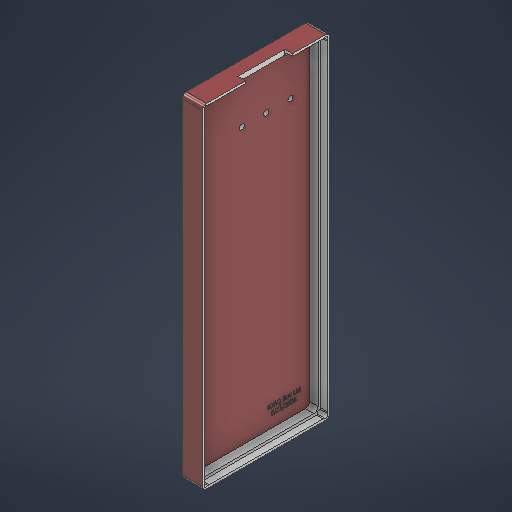
# Autodesk Inventor part: cDAQ_Lid_Box
Saved by Autodesk Inventor 2027 (Build 310192000, 192)
## iProperties
Created: 2026-05-08
Part Number: cDAQ_Lid_Box
Material: Generic
Document SubType Name: Modeling
Designer: giese
Density: 1 g/cm^3
Appearance: Default
Author: giese
Autodesk Inventor part; units mm, degrees
(part 1 of 2)
ref_plane "YZ Plane" through (0, 0, 0) normal (1, 0, 0) x (0, 1, 0)
ref_plane "XZ Plane" through (0, 0, 0) normal (0, 1, 0) x (-1, 0, 0)
ref_plane "XY Plane" through (0, 0, 0) normal (0, 0, 1) x (1, 0, 0)
sketch "Sketch1" plane through (0, 0, 0) normal (1, 0, 0) x (0, 1, 0)
  line L0 (50.7569, 48.4212) -> (-202.6081, 48.4212)
  line L1 (-202.6081, 48.4212) -> (-202.6081, -48.0988)
  line L2 (-202.6081, -48.0988) -> (50.7569, -48.0988)
  line L3 (50.7569, -48.0988) -> (50.7569, 48.4212)
  point P0 (0, 0)
  dimension "d0" = 96.52
  dimension "d1" = 253.365
  constraints: 8 end point, 2 parallel, 1 horizontal, 1 perpendicular
  measures "d0" distance of L2.end L0.start
  measures "d1" distance of L0.start L0.end
extrude "Extrusion1" add sketch "Sketch1" along normal blind 15.24
sketch "Sketch2" plane through (15.24, 0, 0) normal (1, 0, 0) x (0, 0, -1)
  line L0 (-44.6112, 46.9469) -> (44.2888, 46.9469)
  line L1 (44.2888, 46.9469) -> (44.2888, -198.7981)
  line L2 (44.2888, -198.7981) -> (-44.6112, -198.7981)
  line L3 (-44.6112, -198.7981) -> (-44.6112, 46.9469)
  line L4 (-48.4212, 50.7569) -> (-48.4212, -202.6081) projected
  line L5 (-48.4212, -202.6081) -> (48.0988, -202.6081) projected
  point P0 (0, 0)
  dimension "d4" = 88.9
  dimension "d5" = 245.745
  dimension "d6" = 3.81
  dimension "d7" = 3.81
  constraints: 8 end point, 2 parallel, 1 horizontal, 1 perpendicular
  measures "d4" distance of L0.start L0.end
  measures "d5" distance of L0.end L1.end
  measures "d6" distance between parallel lines of L4 L3
  measures "d7" distance between parallel lines of L5 L2
extrude "Extrusion2" cut sketch "Sketch2" against normal blind 11.43
sketch "Sketch3" plane through (0, 0, 0) normal (-1, 0, 0) x (0, 0, 1)
  circle A0 centre (-29.8108, 10.5233) radius 2
  line L0 (-48.0988, -202.6081) -> (-48.0988, 50.7569) projected
  line L1 (-48.0988, 50.7569) -> (48.4212, 50.7569) projected
  circle A1 centre (-11.312, 10.5233) radius 2
  circle A2 centre (7.1869, 10.5233) radius 2
  point P0 (0, 0)
  dimension "d10" = 18.288
  dimension "d11" = 40.2336
  dimension "d12" = 40.2336
  dimension "d13" = 18.4988
  dimension "d14" = 4
  dimension "d15" = 4
  dimension "d16" = 40.2336
  dimension "d17" = 18.4988
  dimension "d18" = 36.9976
  dimension "d21" = 4
  constraints: 3 centre point
  measures "d10" distance from line of L0 A0.centre
  measures "d11" distance from line of L1 A0.centre
  measures "d12" distance from line of L1 A1.centre
  measures "d13" distance of A0.centre A1.centre
  measures "d14" diameter of A1
  measures "d15" diameter of A2
  measures "d16" distance from line of L1 A2.centre
  measures "d17" distance of A1.centre A2.centre
  measures "d18" distance of A0.centre A2.centre
  measures "d21" diameter of A0
extrude "Extrusion3" cut sketch "Sketch3" against normal blind 3.81
sketch "Sketch6" plane through (0, 50.7569, 48.4212) normal (0, 1, 0) x (1, 0, 0)
  line L0 (15.24, 3.81) -> (15.24, 92.71) projected
  line L1 (9.4234, 32.7559) -> (15.24, 32.7559)
  line L2 (15.24, 32.7559) -> (15.24, 68.326)
  line L3 (15.24, 68.326) -> (9.4234, 68.326)
  line L4 (9.4234, 68.326) -> (9.4234, 32.7559)
  line L5 (0, 96.52) -> (15.24, 96.52) projected
  point P0 (0, 48.4212)
  point P1 (12.3317, 68.326)
  point P2 (12.3317, 32.7559)
  dimension "d30" = 5.8166
  dimension "d31" = 35.5701
  dimension "d32" = 28.194
  constraints: 8 end point, 2 midpoint, 2 parallel, 1 horizontal, 1 perpendicular, 1 point on line
  measures "d30" distance between parallel lines of L0 L4
  measures "d31" distance of point (12.332, 68.326) point (12.332, 32.756)
  measures "d32" distance between parallel lines of L5 L3
extrude "Extrusion5" cut sketch "Sketch6" against normal blind 3.81
fillet "Fillet1" radius 3.175 4 edges at (7.62, 50.7569, -48.0988) (7.62, 50.7569, 48.4212) (7.62, -202.6081, 48.4212) (7.62, -202.6081, -48.0988)
sketch "Sketch7" plane through (15.24, 0, 0) normal (1, 0, 0) x (0, 0, -1)
  line L0 (-44.6112, -198.7981) -> (-44.6112, 46.9469) projected
  line L1 (-44.6112, 46.9469) -> (-42.3252, 46.9469)
  line L2 (-42.3252, 48.9469) -> (-46.6112, 48.9469)
  line L3 (-46.6112, 48.9469) -> (-46.6112, 48.4709)
  line L4 (-44.6112, -192.7021) -> (-44.6112, -198.7981)
  line L5 (44.2888, -198.7981) -> (-44.6112, -198.7981) projected
  line L6 (-42.3252, -200.7981) -> (-46.6112, -200.7981)
  line L7 (-46.6112, -200.7981) -> (-46.6112, -192.7021)
  line L8 (44.2888, 46.9469) -> (44.2888, -198.7981) projected
  line L9 (44.2888, -192.7021) -> (44.2888, -198.7981)
  line L10 (44.2888, -198.7981) -> (42.0028, -198.7981)
  line L11 (44.2888, -198.7981) -> (44.2888, -192.7021)
  line L12 (46.2888, -192.7021) -> (46.2888, -200.7981)
  line L13 (46.2888, -200.7981) -> (42.0028, -200.7981)
  line L14 (-44.6112, 46.9469) -> (44.2888, 46.9469) projected
  line L15 (42.0028, 46.9469) -> (44.2888, 46.9469)
  line L16 (46.2888, 48.4709) -> (46.2888, 48.9469)
  line L17 (46.2888, 48.9469) -> (42.0028, 48.9469)
  line L18 (-42.3252, 48.9469) -> (42.0028, 48.9469)
  line L19 (42.0028, 46.9469) -> (-42.3252, 46.9469)
  line L20 (46.2888, 48.4709) -> (46.2888, -192.7021)
  line L21 (44.2888, -192.7021) -> (44.2888, 46.9469)
  line L22 (42.0028, -198.7981) -> (-42.3252, -198.7981)
  line L23 (-42.3252, -200.7981) -> (42.0028, -200.7981)
  line L24 (-46.6112, -192.7021) -> (-46.6112, 48.4709)
  line L25 (-44.6112, 46.9469) -> (-44.6112, -192.7021)
  point P0 (0, 0)
  point P1 (-44.6112, 48.4709)
  point P2 (-44.2302, 48.9789)
  point P3 (44.2888, 48.4709)
  dimension "d10" = 18.288
  dimension "d34" = 2
  dimension "d35" = 2
  dimension "d38" = 2
  dimension "d39" = 2
  dimension "d42" = 2
  dimension "d43" = 2
  dimension "d46" = 2
  dimension "d47" = 2
  constraints: 44 end point, 9 point on line, 4 parallel, 4 perpendicular, 2 collinear, 2 horizontal, 2 vertical
  measures "d34" distance between parallel lines of L2 L1
  measures "d35" distance between parallel lines of L0 L3
  measures "d38" distance between parallel lines of L7 L0
  measures "d39" distance between parallel lines of L5 L6
  measures "d42" distance between parallel lines of L5 L13
  measures "d43" distance between parallel lines of L8 L12
  measures "d46" distance between parallel lines of L14 L17
  measures "d47" distance between parallel lines of L8 L16
extrude "Extrusion6" cut sketch "Sketch7" against normal blind 5
fillet "Fillet2" radius 3.175 8 edges at (12.74, 48.9469, 46.6112) (7.025, 46.9469, 44.6112) (12.74, 48.9469, -46.2888) (7.025, 46.9469, -44.2888) (7.025, -198.7981, 44.6112) (12.74, -200.7981, 46.6112) (7.025, -198.7981, -44.2888) (12.74, -200.7981, -46.2888)
sketch "Sketch11" plane through (10.24, 0, 0) normal (1, 0, 0) x (0, 0, -1)
  circle A0 centre (45.1266, 48.0137) radius 1.5
  line L0 (44.9238, 50.7569) -> (19.9048, 50.7569) projected
  line L1 (48.0988, -199.4331) -> (48.0988, 47.5819) projected
  arc A1 (46.2888, 45.7719) -> (43.1138, 48.9469) centre (43.1138, 45.7719) ccw projected
  circle A2 centre (-45.678, 48.0137) radius 1.5
  line L2 (-48.4212, 47.5819) -> (-48.4212, -199.4331) projected
  line L3 (-15.6653, 50.7569) -> (-45.2462, 50.7569) projected
  circle A3 centre (45.3556, -199.8649) radius 1.5
  line L4 (-45.2462, -202.6081) -> (44.9238, -202.6081) projected
  circle A4 centre (-45.678, -199.8649) radius 1.5
  point P0 (0, 0)
  point P1 (45.3589, 48.017)
  dimension "d56" = 2.7432
  dimension "d57" = 2.7399
  dimension "d58" = 3
  dimension "d59" = 2.7432
  dimension "d60" = 2.7432
  dimension "d61" = 3
  dimension "d62" = 3
  dimension "d63" = 2.7432
  dimension "d64" = 2.7432
  dimension "d65" = 3
  dimension "d66" = 2.7432
  dimension "d67" = 2.7432
  constraints: 4 centre point, 1 point on circle
  measures "d56" distance from line of L0 A0.centre
  measures "d57" distance from line of L1 point (45.359, 48.017)
  measures "d58" diameter of A0
  measures "d59" distance from line of L2 A2.centre
  measures "d60" distance from line of L3 A2.centre
  measures "d61" diameter of A2
  measures "d62" diameter of A3
  measures "d63" distance from line of L1 A3.centre
  measures "d64" distance from line of L4 A3.centre
  measures "d65" diameter of A4
  measures "d66" distance from line of L2 A4.centre
  measures "d67" distance from line of L4 A4.centre
extrude "Extrusion8" cut sketch "Sketch11" along normal blind 5.08 and the other way blind 10.414
sketch "Sketch13" plane through (3.81, 0, 0) normal (1, 0, 0) x (0, 0, -1)
  line L0 (12.2621, -182.3354) -> (37.3179, -182.3354) construction
  line L1 (37.3179, -182.3354) -> (37.3179, -191.1997) construction
  line L2 (37.3179, -191.1997) -> (12.2621, -191.1997) construction
  line L3 (12.2621, -191.1997) -> (12.2621, -182.3354) construction
  spline S0 degree 2 poles (13.4502, -185.5711) (13.213, -185.5711) (12.8203, -185.4254) (12.6795, -185.2772) knots 0 0 0 1 2 2 2
  spline S1 degree 2 poles (12.6795, -185.2772) (12.5387, -185.1315) (12.3831, -184.6819) (12.3831, -184.3806) knots 0 0 0 1 2 2 2
  spline S2 degree 2 poles (12.3831, -184.3806) (12.3831, -184.0792) (12.5437, -183.6396) (12.6795, -183.4914) knots 0 0 0 1 2 2 2
  spline S3 degree 2 poles (12.6795, -183.4914) (12.8154, -183.3407) (13.218, -183.1801) (13.4502, -183.1801) knots 0 0 0 1 2 2 2
  spline S4 degree 2 poles (13.4502, -183.1801) (13.6379, -183.1801) (13.9886, -183.2864) (14.1245, -183.3555) knots 0 0 0 1 2 2 2
  line L4 (14.1245, -183.3555) -> (14.1245, -183.7878)
  line L5 (14.1245, -183.7878) -> (14.1022, -183.7878)
  spline S5 degree 2 poles (14.1022, -183.7878) (14.0602, -183.7532) (13.9318, -183.6643) (13.8404, -183.6173) knots 0 0 0 1 2 2 2
  spline S6 degree 2 poles (13.8404, -183.6173) (13.7589, -183.5778) (13.5415, -183.5161) (13.4427, -183.5161) knots 0 0 0 1 2 2 2
  spline S7 degree 2 poles (13.4427, -183.5161) (13.1439, -183.5161) (12.7808, -183.9681) (12.7808, -184.3806) knots 0 0 0 1 2 2 2
  spline S8 degree 2 poles (12.7808, -184.3806) (12.7808, -184.7832) (13.1315, -185.2352) (13.4427, -185.2352) knots 0 0 0 1 2 2 2
  spline S9 degree 2 poles (13.4427, -185.2352) (13.6305, -185.2352) (13.9713, -185.0796) (14.1022, -184.9586) knots 0 0 0 1 2 2 2
  line L6 (14.1022, -184.9586) -> (14.1245, -184.9586)
  line L7 (14.1245, -184.9586) -> (14.1245, -185.3908)
  spline S10 degree 2 poles (14.1245, -185.3908) (14.0677, -185.418) (13.8948, -185.4945) (13.8256, -185.5118) knots 0 0 0 1 2 2 2
  spline S11 degree 2 poles (13.8256, -185.5118) (13.7268, -185.5415) (13.5712, -185.5711) (13.4502, -185.5711) knots 0 0 0 1 2 2 2
  spline S12 degree 2 poles (16.9082, -183.9977) (16.9082, -184.4152) (16.5698, -185.087) (16.2857, -185.2747) knots 0 0 0 1 2 2 2
  spline S13 degree 2 poles (16.2857, -185.2747) (16.0536, -185.4204) (15.5768, -185.5192) (15.2063, -185.5192) knots 0 0 0 1 2 2 2
  line L8 (15.2063, -185.5192) -> (14.5049, -185.5192)
  line L9 (14.5049, -185.5192) -> (14.5049, -182.4712)
  line L10 (14.5049, -182.4712) -> (15.1989, -182.4712)
  spline S14 degree 2 poles (15.1989, -182.4712) (15.6287, -182.4712) (16.1178, -182.5997) (16.2907, -182.7133) knots 0 0 0 1 2 2 2
  spline S15 degree 2 poles (16.2907, -182.7133) (16.5846, -182.9084) (16.9082, -183.5531) (16.9082, -183.9977) knots 0 0 0 1 2 2 2
  spline S16 degree 2 poles (16.4858, -183.9928) (16.4858, -183.642) (16.2536, -183.1456) (16.0239, -183.0048) knots 0 0 0 1 2 2 2
  spline S17 degree 2 poles (16.0239, -183.0048) (15.8609, -182.9084) (15.4929, -182.822) (15.2187, -182.822) knots 0 0 0 1 2 2 2
  line L11 (15.2187, -182.822) -> (14.9099, -182.822)
  line L12 (14.9099, -182.822) -> (14.9099, -185.1685)
  line L13 (14.9099, -185.1685) -> (15.2187, -185.1685)
  spline S18 degree 2 poles (15.2187, -185.1685) (15.4879, -185.1685) (15.8955, -185.0821) (16.061, -184.966) knots 0 0 0 1 2 2 2
  spline S19 degree 2 poles (16.061, -184.966) (16.2734, -184.8227) (16.4858, -184.3485) (16.4858, -183.9928) knots 0 0 0 1 2 2 2
  line L14 (17.0193, -185.5192) -> (18.0469, -182.4712)
  line L15 (18.0469, -182.4712) -> (18.5458, -182.4712)
  line L16 (18.5458, -182.4712) -> (19.5733, -185.5192)
  line L17 (19.5733, -185.5192) -> (19.146, -185.5192)
  line L18 (19.146, -185.5192) -> (18.8694, -184.6671)
  line L19 (18.8694, -184.6671) -> (17.706, -184.6671)
  line L20 (17.706, -184.6671) -> (17.4294, -185.5192)
  line L21 (17.4294, -185.5192) -> (17.0193, -185.5192)
  line L22 (18.7582, -184.3213) -> (18.2864, -182.8862)
  line L23 (18.2864, -182.8862) -> (17.8171, -184.3213)
  line L24 (17.8171, -184.3213) -> (18.7582, -184.3213)
  spline S20 degree 2 poles (22.3941, -186.2652) (22.2829, -186.2924) (22.0409, -186.322) (21.9198, -186.322) knots 0 0 0 1 2 2 2
  spline S21 degree 2 poles (21.9198, -186.322) (21.5765, -186.322) (21.1492, -185.9392) (21.1294, -185.5835) knots 0 0 0 1 2 2 2
  spline S22 degree 2 poles (21.1294, -185.5835) (21.1023, -185.5835) (21.0553, -185.5835) (21.0356, -185.5835) knots 0 0 0 1 2 2 2
  spline S23 degree 2 poles (21.0356, -185.5835) (20.7268, -185.5835) (20.2303, -185.3735) (20.0525, -185.1685) knots 0 0 0 1 2 2 2
  spline S24 degree 2 poles (20.0525, -185.1685) (19.8771, -184.966) (19.6894, -184.3732) (19.6894, -183.9977) knots 0 0 0 1 2 2 2
  spline S25 degree 2 poles (19.6894, -183.9977) (19.6894, -183.6124) (19.8796, -183.0295) (20.055, -182.822) knots 0 0 0 1 2 2 2
  spline S26 degree 2 poles (20.055, -182.822) (20.2328, -182.617) (20.7293, -182.407) (21.0356, -182.407) knots 0 0 0 1 2 2 2
  spline S27 degree 2 poles (21.0356, -182.407) (21.3468, -182.407) (21.8457, -182.6244) (22.0186, -182.822) knots 0 0 0 1 2 2 2
  spline S28 degree 2 poles (22.0186, -182.822) (22.1915, -183.0221) (22.3842, -183.6173) (22.3842, -183.9977) knots 0 0 0 1 2 2 2
  spline S29 degree 2 poles (22.3842, -183.9977) (22.3842, -184.5905) (21.9223, -185.3612) (21.5197, -185.497) knots 0 0 0 1 2 2 2
  spline S30 degree 2 poles (21.5197, -185.497) (21.5296, -185.6106) (21.5889, -185.7934) (21.6358, -185.8453) knots 0 0 0 1 2 2 2
  spline S31 degree 2 poles (21.6358, -185.8453) (21.6926, -185.9095) (21.8482, -185.9688) (21.9865, -185.9688) knots 0 0 0 1 2 2 2
  spline S32 degree 2 poles (21.9865, -185.9688) (22.068, -185.9688) (22.2903, -185.9169) (22.3397, -185.8972) knots 0 0 0 1 2 2 2
  line L25 (22.3397, -185.8972) -> (22.3941, -185.8972)
  line L26 (22.3941, -185.8972) -> (22.3941, -186.2652)
  spline S33 degree 2 poles (21.9618, -183.9977) (21.9618, -183.6939) (21.8309, -183.2271) (21.7124, -183.0739) knots 0 0 0 1 2 2 2
  spline S34 degree 2 poles (21.7124, -183.0739) (21.5913, -182.9159) (21.2505, -182.7578) (21.038, -182.7578) knots 0 0 0 1 2 2 2
  spline S35 degree 2 poles (21.038, -182.7578) (20.8182, -182.7578) (20.4872, -182.9109) (20.3613, -183.0739) knots 0 0 0 1 2 2 2
  spline S36 degree 2 poles (20.3613, -183.0739) (20.2402, -183.2295) (20.1118, -183.7013) (20.1118, -183.9977) knots 0 0 0 1 2 2 2
  spline S37 degree 2 poles (20.1118, -183.9977) (20.1118, -184.5979) (20.6157, -185.2377) (21.038, -185.2377) knots 0 0 0 1 2 2 2
  spline S38 degree 2 poles (21.038, -185.2377) (21.4604, -185.2377) (21.9618, -184.5979) (21.9618, -183.9977) knots 0 0 0 1 2 2 2
  spline S39 degree 2 poles (26.2053, -184.5831) (26.2053, -184.8104) (26.0324, -185.1586) (25.8892, -185.2722) knots 0 0 0 1 2 2 2
  spline S40 degree 2 poles (25.8892, -185.2722) (25.7163, -185.4056) (25.3235, -185.5192) (25.0123, -185.5192) knots 0 0 0 1 2 2 2
  line L27 (25.0123, -185.5192) -> (24.1379, -185.5192)
  line L28 (24.1379, -185.5192) -> (24.1379, -182.4712)
  line L29 (24.1379, -182.4712) -> (24.9456, -182.4712)
  spline S41 degree 2 poles (24.9456, -182.4712) (25.2717, -182.4712) (25.5977, -182.5132) (25.7459, -182.5948) knots 0 0 0 1 2 2 2
  spline S42 degree 2 poles (25.7459, -182.5948) (25.9114, -182.6812) (26.0621, -182.9653) (26.0621, -183.1579) knots 0 0 0 1 2 2 2
  spline S43 degree 2 poles (26.0621, -183.1579) (26.0621, -183.3728) (25.8348, -183.7137) (25.6347, -183.81) knots 0 0 0 1 2 2 2
  line L30 (25.6347, -183.81) -> (25.6347, -183.8248)
  spline S44 degree 2 poles (25.6347, -183.8248) (25.9064, -183.8989) (26.2053, -184.2917) (26.2053, -184.5831) knots 0 0 0 1 2 2 2
  spline S45 degree 2 poles (25.7829, -184.6004) (25.7829, -184.4275) (25.6841, -184.2052) (25.5359, -184.1262) knots 0 0 0 1 2 2 2
  spline S46 degree 2 poles (25.5359, -184.1262) (25.4396, -184.0768) (25.2124, -184.0471) (25.0024, -184.0471) knots 0 0 0 1 2 2 2
  line L31 (25.0024, -184.0471) -> (24.543, -184.0471)
  line L32 (24.543, -184.0471) -> (24.543, -185.1734)
  line L33 (24.543, -185.1734) -> (24.8715, -185.1734)
  spline S47 degree 2 poles (24.8715, -185.1734) (25.1383, -185.1734) (25.4446, -185.124) (25.5631, -185.045) knots 0 0 0 1 2 2 2
  spline S48 degree 2 poles (25.5631, -185.045) (25.6767, -184.9635) (25.7829, -184.761) (25.7829, -184.6004) knots 0 0 0 1 2 2 2
  spline S49 degree 2 poles (25.6397, -183.2147) (25.6397, -183.106) (25.5656, -182.943) (25.4841, -182.8961) knots 0 0 0 1 2 2 2
  spline S50 degree 2 poles (25.4841, -182.8961) (25.3853, -182.8418) (25.1457, -182.8171) (24.9308, -182.8171) knots 0 0 0 1 2 2 2
  line L34 (24.9308, -182.8171) -> (24.543, -182.8171)
  line L35 (24.543, -182.8171) -> (24.543, -183.7087)
  line L36 (24.543, -183.7087) -> (25.0024, -183.7087)
  spline S51 degree 2 poles (25.0024, -183.7087) (25.1926, -183.7087) (25.3729, -183.6692) (25.4693, -183.6075) knots 0 0 0 1 2 2 2
  spline S52 degree 2 poles (25.4693, -183.6075) (25.5631, -183.5482) (25.6397, -183.358) (25.6397, -183.2147) knots 0 0 0 1 2 2 2
  spline S53 degree 2 poles (28.458, -184.3756) (28.458, -184.9536) (27.9022, -185.5835) (27.4379, -185.5835) knots 0 0 0 1 2 2 2
  spline S54 degree 2 poles (27.4379, -185.5835) (26.9611, -185.5835) (26.4153, -184.9339) (26.4153, -184.3756) knots 0 0 0 1 2 2 2
  spline S55 degree 2 poles (26.4153, -184.3756) (26.4153, -183.8026) (26.9784, -183.1678) (27.4379, -183.1678) knots 0 0 0 1 2 2 2
  spline S56 degree 2 poles (27.4379, -183.1678) (27.9022, -183.1678) (28.458, -183.8001) (28.458, -184.3756) knots 0 0 0 1 2 2 2
  spline S57 degree 2 poles (28.0603, -184.3756) (28.0603, -183.931) (27.7367, -183.4988) (27.4379, -183.4988) knots 0 0 0 1 2 2 2
  spline S58 degree 2 poles (27.4379, -183.4988) (27.139, -183.4988) (26.8129, -183.931) (26.8129, -184.3756) knots 0 0 0 1 2 2 2
  spline S59 degree 2 poles (26.8129, -184.3756) (26.8129, -184.8079) (27.139, -185.2525) (27.4379, -185.2525) knots 0 0 0 1 2 2 2
  spline S60 degree 2 poles (27.4379, -185.2525) (27.7343, -185.2525) (28.0603, -184.8153) (28.0603, -184.3756) knots 0 0 0 1 2 2 2
  line L37 (30.6291, -185.5192) -> (30.1573, -185.5192)
  line L38 (30.1573, -185.5192) -> (29.6016, -184.6597)
  line L39 (29.6016, -184.6597) -> (29.031, -185.5192)
  line L40 (29.031, -185.5192) -> (28.5938, -185.5192)
  line L41 (28.5938, -185.5192) -> (29.3867, -184.3855)
  line L42 (29.3867, -184.3855) -> (28.6012, -183.232)
  line L43 (28.6012, -183.232) -> (29.073, -183.232)
  line L44 (29.073, -183.232) -> (29.6263, -184.0842)
  line L45 (29.6263, -184.0842) -> (30.1919, -183.232)
  line L46 (30.1919, -183.232) -> (30.6291, -183.232)
  line L47 (30.6291, -183.232) -> (29.8412, -184.3608)
  line L48 (29.8412, -184.3608) -> (30.6291, -185.5192)
  line L49 (34.0328, -185.5192) -> (32.2667, -185.5192)
  line L50 (32.2667, -185.5192) -> (32.2667, -182.4712)
  line L51 (32.2667, -182.4712) -> (32.6718, -182.4712)
  line L52 (32.6718, -182.4712) -> (32.6718, -185.1586)
  line L53 (32.6718, -185.1586) -> (34.0328, -185.1586)
  line L54 (34.0328, -185.1586) -> (34.0328, -185.5192)
  line L55 (34.7145, -185.5192) -> (34.3292, -185.5192)
  line L56 (34.3292, -185.5192) -> (34.3292, -183.232)
  line L57 (34.3292, -183.232) -> (34.7145, -183.232)
  line L58 (34.7145, -183.232) -> (34.7145, -185.5192)
  line L59 (34.7417, -182.8516) -> (34.3045, -182.8516)
  line L60 (34.3045, -182.8516) -> (34.3045, -182.4515)
  line L61 (34.3045, -182.4515) -> (34.7417, -182.4515)
  line L62 (34.7417, -182.4515) -> (34.7417, -182.8516)
  line L63 (37.0388, -185.5192) -> (36.6535, -185.5192)
  line L64 (36.6535, -185.5192) -> (36.6535, -185.2871)
  spline S61 degree 2 poles (36.6535, -185.2871) (36.5646, -185.3612) (36.4337, -185.46) (36.3447, -185.502) knots 0 0 0 1 2 2 2
  spline S62 degree 2 poles (36.3447, -185.502) (36.2632, -185.5415) (36.0879, -185.5835) (35.9718, -185.5835) knots 0 0 0 1 2 2 2
  spline S63 degree 2 poles (35.9718, -185.5835) (35.784, -185.5835) (35.4679, -185.4279) (35.3567, -185.2772) knots 0 0 0 1 2 2 2
  spline S64 degree 2 poles (35.3567, -185.2772) (35.2456, -185.1265) (35.1221, -184.6819) (35.1221, -184.3929) knots 0 0 0 1 2 2 2
  spline S65 degree 2 poles (35.1221, -184.3929) (35.1221, -184.0916) (35.2777, -183.6519) (35.4135, -183.4864) knots 0 0 0 1 2 2 2
  spline S66 degree 2 poles (35.4135, -183.4864) (35.5395, -183.3382) (35.8927, -183.1678) (36.0879, -183.1678) knots 0 0 0 1 2 2 2
  spline S67 degree 2 poles (36.0879, -183.1678) (36.2583, -183.1678) (36.5127, -183.2444) (36.6535, -183.3234) knots 0 0 0 1 2 2 2
  line L65 (36.6535, -183.3234) -> (36.6535, -182.3354)
  line L66 (36.6535, -182.3354) -> (37.0388, -182.3354)
  line L67 (37.0388, -182.3354) -> (37.0388, -185.5192)
  line L68 (36.6535, -184.9635) -> (36.6535, -183.642)
  spline S68 degree 2 poles (36.6535, -183.642) (36.5102, -183.5729) (36.283, -183.521) (36.1521, -183.521) knots 0 0 0 1 2 2 2
  spline S69 degree 2 poles (36.1521, -183.521) (35.8557, -183.521) (35.5197, -183.9656) (35.5197, -184.3855) knots 0 0 0 1 2 2 2
  spline S70 degree 2 poles (35.5197, -184.3855) (35.5197, -184.7906) (35.7766, -185.2179) (36.0607, -185.2179) knots 0 0 0 1 2 2 2
  spline S71 degree 2 poles (36.0607, -185.2179) (36.2114, -185.2179) (36.5176, -185.0796) (36.6535, -184.9635) knots 0 0 0 1 2 2 2
  spline S72 degree 2 poles (17.2515, -189.5695) (17.2515, -189.7893) (17.1107, -190.1647) (16.9823, -190.303) knots 0 0 0 1 2 2 2
  spline S73 degree 2 poles (16.9823, -190.303) (16.8538, -190.4414) (16.471, -190.6019) (16.2339, -190.6019) knots 0 0 0 1 2 2 2
  spline S74 degree 2 poles (16.2339, -190.6019) (16.0165, -190.6019) (15.5917, -190.5056) (15.436, -190.429) knots 0 0 0 1 2 2 2
  line L69 (15.436, -190.429) -> (15.436, -189.9968)
  line L70 (15.436, -189.9968) -> (15.4657, -189.9968)
  spline S75 degree 2 poles (15.4657, -189.9968) (15.5126, -190.0313) (15.688, -190.1203) (15.7942, -190.1598) knots 0 0 0 1 2 2 2
  spline S76 degree 2 poles (15.7942, -190.1598) (15.9152, -190.2018) (16.1153, -190.2487) (16.2413, -190.2487) knots 0 0 0 1 2 2 2
  spline S77 degree 2 poles (16.2413, -190.2487) (16.3648, -190.2487) (16.597, -190.1598) (16.6809, -190.0635) knots 0 0 0 1 2 2 2
  spline S78 degree 2 poles (16.6809, -190.0635) (16.7575, -189.9721) (16.8365, -189.73) (16.8365, -189.567) knots 0 0 0 1 2 2 2
  spline S79 degree 2 poles (16.8365, -189.567) (16.8365, -189.404) (16.7476, -189.1965) (16.6636, -189.1273) knots 0 0 0 1 2 2 2
  spline S80 degree 2 poles (16.6636, -189.1273) (16.5772, -189.0508) (16.3203, -188.9865) (16.1647, -188.9865) knots 0 0 0 1 2 2 2
  spline S81 degree 2 poles (16.1647, -188.9865) (15.9967, -188.9865) (15.6633, -189.0384) (15.562, -189.0606) knots 0 0 0 1 2 2 2
  line L71 (15.562, -189.0606) -> (15.562, -187.4897)
  line L72 (15.562, -187.4897) -> (17.2342, -187.4897)
  line L73 (17.2342, -187.4897) -> (17.2342, -187.8479)
  line L74 (17.2342, -187.8479) -> (15.9548, -187.8479)
  line L75 (15.9548, -187.8479) -> (15.9548, -188.6605)
  spline S82 degree 2 poles (15.9548, -188.6605) (16.0289, -188.6506) (16.1721, -188.6432) (16.2314, -188.6432) knots 0 0 0 1 2 2 2
  spline S83 degree 2 poles (16.2314, -188.6432) (16.466, -188.6432) (16.7896, -188.7198) (16.9378, -188.8334) knots 0 0 0 1 2 2 2
  spline S84 degree 2 poles (16.9378, -188.8334) (17.0885, -188.947) (17.2515, -189.2928) (17.2515, -189.5695) knots 0 0 0 1 2 2 2
  line L76 (18.9583, -187.3539) -> (17.7653, -191.1997)
  line L77 (17.7653, -191.1997) -> (17.4195, -191.1997)
  line L78 (17.4195, -191.1997) -> (18.6075, -187.3539)
  line L79 (18.6075, -187.3539) -> (18.9583, -187.3539)
  line L80 (21.1739, -190.5377) -> (19.2942, -190.5377)
  line L81 (19.2942, -190.5377) -> (19.2942, -190.1054)
  spline S85 degree 2 poles (19.2942, -190.1054) (19.4968, -189.9153) (19.8574, -189.562) (20.0303, -189.3719) knots 0 0 0 1 2 2 2
  spline S86 degree 2 poles (20.0303, -189.3719) (20.3786, -188.989) (20.633, -188.5296) (20.633, -188.285) knots 0 0 0 1 2 2 2
  spline S87 degree 2 poles (20.633, -188.285) (20.633, -188.1566) (20.5539, -187.9639) (20.4823, -187.9022) knots 0 0 0 1 2 2 2
  spline S88 degree 2 poles (20.4823, -187.9022) (20.4107, -187.8404) (20.2229, -187.7787) (20.1093, -187.7787) knots 0 0 0 1 2 2 2
  spline S89 degree 2 poles (20.1093, -187.7787) (20.0006, -187.7787) (19.7783, -187.833) (19.6771, -187.875) knots 0 0 0 1 2 2 2
  spline S90 degree 2 poles (19.6771, -187.875) (19.5906, -187.9096) (19.4301, -188.0084) (19.3807, -188.043) knots 0 0 0 1 2 2 2
  line L82 (19.3807, -188.043) -> (19.3584, -188.043)
  line L83 (19.3584, -188.043) -> (19.3584, -187.6083)
  spline S91 degree 2 poles (19.3584, -187.6083) (19.4844, -187.5465) (19.9364, -187.4255) (20.139, -187.4255) knots 0 0 0 1 2 2 2
  spline S92 degree 2 poles (20.139, -187.4255) (20.5663, -187.4255) (21.0479, -187.8775) (21.0479, -188.2628) knots 0 0 0 1 2 2 2
  spline S93 degree 2 poles (21.0479, -188.2628) (21.0479, -188.4431) (20.9639, -188.7445) (20.8898, -188.8729) knots 0 0 0 1 2 2 2
  spline S94 degree 2 poles (20.8898, -188.8729) (20.8157, -189.0063) (20.6009, -189.2681) (20.4823, -189.3941) knots 0 0 0 1 2 2 2
  spline S95 degree 2 poles (20.4823, -189.3941) (20.2896, -189.604) (19.8179, -190.0536) (19.6771, -190.1845) knots 0 0 0 1 2 2 2
  line L84 (19.6771, -190.1845) -> (21.1739, -190.1845)
  line L85 (21.1739, -190.1845) -> (21.1739, -190.5377)
  line L86 (23.308, -190.5377) -> (21.821, -190.5377)
  line L87 (21.821, -190.5377) -> (21.821, -190.2265)
  line L88 (21.821, -190.2265) -> (22.3743, -190.2265)
  line L89 (22.3743, -190.2265) -> (22.3743, -188.1838)
  line L90 (22.3743, -188.1838) -> (21.821, -188.1838)
  line L91 (21.821, -188.1838) -> (21.821, -187.9047)
  spline S96 degree 2 poles (21.821, -187.9047) (22.1347, -187.9047) (22.4311, -187.7268) (22.4509, -187.4798) knots 0 0 0 1 2 2 2
  line L92 (22.4509, -187.4798) -> (22.7671, -187.4798)
  line L93 (22.7671, -187.4798) -> (22.7671, -190.2265)
  line L94 (22.7671, -190.2265) -> (23.308, -190.2265)
  line L95 (23.308, -190.2265) -> (23.308, -190.5377)
  line L96 (25.1358, -187.3539) -> (23.9428, -191.1997)
  line L97 (23.9428, -191.1997) -> (23.597, -191.1997)
  line L98 (23.597, -191.1997) -> (24.7851, -187.3539)
  line L99 (24.7851, -187.3539) -> (25.1358, -187.3539)
  line L100 (27.3514, -190.5377) -> (25.4717, -190.5377)
  line L101 (25.4717, -190.5377) -> (25.4717, -190.1054)
  spline S97 degree 2 poles (25.4717, -190.1054) (25.6743, -189.9153) (26.0349, -189.562) (26.2078, -189.3719) knots 0 0 0 1 2 2 2
  spline S98 degree 2 poles (26.2078, -189.3719) (26.5561, -188.989) (26.8105, -188.5296) (26.8105, -188.285) knots 0 0 0 1 2 2 2
  spline S99 degree 2 poles (26.8105, -188.285) (26.8105, -188.1566) (26.7314, -187.9639) (26.6598, -187.9022) knots 0 0 0 1 2 2 2
  spline S100 degree 2 poles (26.6598, -187.9022) (26.5882, -187.8404) (26.4004, -187.7787) (26.2868, -187.7787) knots 0 0 0 1 2 2 2
  spline S101 degree 2 poles (26.2868, -187.7787) (26.1781, -187.7787) (25.9558, -187.833) (25.8546, -187.875) knots 0 0 0 1 2 2 2
  spline S102 degree 2 poles (25.8546, -187.875) (25.7681, -187.9096) (25.6076, -188.0084) (25.5582, -188.043) knots 0 0 0 1 2 2 2
  line L102 (25.5582, -188.043) -> (25.5359, -188.043)
  line L103 (25.5359, -188.043) -> (25.5359, -187.6083)
  spline S103 degree 2 poles (25.5359, -187.6083) (25.6619, -187.5465) (26.1139, -187.4255) (26.3165, -187.4255) knots 0 0 0 1 2 2 2
  spline S104 degree 2 poles (26.3165, -187.4255) (26.7438, -187.4255) (27.2254, -187.8775) (27.2254, -188.2628) knots 0 0 0 1 2 2 2
  spline S105 degree 2 poles (27.2254, -188.2628) (27.2254, -188.4431) (27.1415, -188.7445) (27.0674, -188.8729) knots 0 0 0 1 2 2 2
  spline S106 degree 2 poles (27.0674, -188.8729) (26.9933, -189.0063) (26.7784, -189.2681) (26.6598, -189.3941) knots 0 0 0 1 2 2 2
  spline S107 degree 2 poles (26.6598, -189.3941) (26.4671, -189.604) (25.9954, -190.0536) (25.8546, -190.1845) knots 0 0 0 1 2 2 2
  line L104 (25.8546, -190.1845) -> (27.3514, -190.1845)
  line L105 (27.3514, -190.1845) -> (27.3514, -190.5377)
  spline S108 degree 2 poles (29.6559, -189.0137) (29.6559, -189.8337) (29.1792, -190.6019) (28.6827, -190.6019) knots 0 0 0 1 2 2 2
  spline S109 degree 2 poles (28.6827, -190.6019) (28.1789, -190.6019) (27.7071, -189.8189) (27.7071, -189.0162) knots 0 0 0 1 2 2 2
  spline S110 degree 2 poles (27.7071, -189.0162) (27.7071, -188.1912) (28.1838, -187.428) (28.6827, -187.428) knots 0 0 0 1 2 2 2
  spline S111 degree 2 poles (28.6827, -187.428) (29.1842, -187.428) (29.6559, -188.2184) (29.6559, -189.0137) knots 0 0 0 1 2 2 2
  spline S112 degree 2 poles (29.1323, -189.9424) (29.1916, -189.7918) (29.241, -189.3274) (29.241, -189.0137) knots 0 0 0 1 2 2 2
  spline S113 degree 2 poles (29.241, -189.0137) (29.241, -188.7) (29.1916, -188.2381) (29.1298, -188.0825) knots 0 0 0 1 2 2 2
  spline S114 degree 2 poles (29.1298, -188.0825) (29.0681, -187.9269) (28.8532, -187.7663) (28.6827, -187.7663) knots 0 0 0 1 2 2 2
  spline S115 degree 2 poles (28.6827, -187.7663) (28.5123, -187.7663) (28.2925, -187.9269) (28.2283, -188.0874) knots 0 0 0 1 2 2 2
  spline S116 degree 2 poles (28.2283, -188.0874) (28.1665, -188.2431) (28.1221, -188.7173) (28.1221, -189.0162) knots 0 0 0 1 2 2 2
  spline S117 degree 2 poles (28.1221, -189.0162) (28.1221, -189.3373) (28.1616, -189.7671) (28.2258, -189.935) knots 0 0 0 1 2 2 2
  spline S118 degree 2 poles (28.2258, -189.935) (28.2851, -190.0931) (28.5049, -190.2635) (28.6827, -190.2635) knots 0 0 0 1 2 2 2
  spline S119 degree 2 poles (28.6827, -190.2635) (28.8507, -190.2635) (29.0705, -190.103) (29.1323, -189.9424) knots 0 0 0 1 2 2 2
  line L106 (31.9259, -190.5377) -> (30.0462, -190.5377)
  line L107 (30.0462, -190.5377) -> (30.0462, -190.1054)
  spline S120 degree 2 poles (30.0462, -190.1054) (30.2487, -189.9153) (30.6094, -189.562) (30.7823, -189.3719) knots 0 0 0 1 2 2 2
  spline S121 degree 2 poles (30.7823, -189.3719) (31.1305, -188.989) (31.3849, -188.5296) (31.3849, -188.285) knots 0 0 0 1 2 2 2
  spline S122 degree 2 poles (31.3849, -188.285) (31.3849, -188.1566) (31.3059, -187.9639) (31.2343, -187.9022) knots 0 0 0 1 2 2 2
  spline S123 degree 2 poles (31.2343, -187.9022) (31.1626, -187.8404) (30.9749, -187.7787) (30.8613, -187.7787) knots 0 0 0 1 2 2 2
  spline S124 degree 2 poles (30.8613, -187.7787) (30.7526, -187.7787) (30.5303, -187.833) (30.429, -187.875) knots 0 0 0 1 2 2 2
  spline S125 degree 2 poles (30.429, -187.875) (30.3426, -187.9096) (30.182, -188.0084) (30.1326, -188.043) knots 0 0 0 1 2 2 2
  line L108 (30.1326, -188.043) -> (30.1104, -188.043)
  line L109 (30.1104, -188.043) -> (30.1104, -187.6083)
  spline S126 degree 2 poles (30.1104, -187.6083) (30.2364, -187.5465) (30.6884, -187.4255) (30.8909, -187.4255) knots 0 0 0 1 2 2 2
  spline S127 degree 2 poles (30.8909, -187.4255) (31.3183, -187.4255) (31.7999, -187.8775) (31.7999, -188.2628) knots 0 0 0 1 2 2 2
  spline S128 degree 2 poles (31.7999, -188.2628) (31.7999, -188.4431) (31.7159, -188.7445) (31.6418, -188.8729) knots 0 0 0 1 2 2 2
  spline S129 degree 2 poles (31.6418, -188.8729) (31.5677, -189.0063) (31.3528, -189.2681) (31.2343, -189.3941) knots 0 0 0 1 2 2 2
  spline S130 degree 2 poles (31.2343, -189.3941) (31.0416, -189.604) (30.5698, -190.0536) (30.429, -190.1845) knots 0 0 0 1 2 2 2
  line L110 (30.429, -190.1845) -> (31.9259, -190.1845)
  line L111 (31.9259, -190.1845) -> (31.9259, -190.5377)
  spline S131 degree 2 poles (34.26, -189.5497) (34.26, -189.7843) (34.1044, -190.182) (33.9735, -190.3154) knots 0 0 0 1 2 2 2
  spline S132 degree 2 poles (33.9735, -190.3154) (33.8377, -190.4562) (33.4968, -190.6019) (33.2918, -190.6019) knots 0 0 0 1 2 2 2
  spline S133 degree 2 poles (33.2918, -190.6019) (33.0868, -190.6019) (32.7484, -190.4636) (32.62, -190.3253) knots 0 0 0 1 2 2 2
  spline S134 degree 2 poles (32.62, -190.3253) (32.4619, -190.1598) (32.284, -189.604) (32.284, -189.199) knots 0 0 0 1 2 2 2
  spline S135 degree 2 poles (32.284, -189.199) (32.284, -188.8013) (32.447, -188.1615) (32.6175, -187.9244) knots 0 0 0 1 2 2 2
  spline S136 degree 2 poles (32.6175, -187.9244) (32.783, -187.6922) (33.3066, -187.4329) (33.6499, -187.4329) knots 0 0 0 1 2 2 2
  spline S137 degree 2 poles (33.6499, -187.4329) (33.7512, -187.4329) (33.9291, -187.4527) (33.9957, -187.4749) knots 0 0 0 1 2 2 2
  line L112 (33.9957, -187.4749) -> (33.9957, -187.8676)
  line L113 (33.9957, -187.8676) -> (33.9785, -187.8676)
  spline S138 degree 2 poles (33.9785, -187.8676) (33.9216, -187.838) (33.7142, -187.7861) (33.5956, -187.7861) knots 0 0 0 1 2 2 2
  spline S139 degree 2 poles (33.5956, -187.7861) (33.2152, -187.7861) (32.7484, -188.2999) (32.7039, -188.8037) knots 0 0 0 1 2 2 2
  spline S140 degree 2 poles (32.7039, -188.8037) (32.8497, -188.7025) (33.1559, -188.5913) (33.3387, -188.5913) knots 0 0 0 1 2 2 2
  spline S141 degree 2 poles (33.3387, -188.5913) (33.5166, -188.5913) (33.7833, -188.663) (33.9291, -188.7716) knots 0 0 0 1 2 2 2
  spline S142 degree 2 poles (33.9291, -188.7716) (34.097, -188.8976) (34.26, -189.2879) (34.26, -189.5497) knots 0 0 0 1 2 2 2
  spline S143 degree 2 poles (33.8451, -189.567) (33.8451, -189.3793) (33.7463, -189.1249) (33.6376, -189.0359) knots 0 0 0 1 2 2 2
  spline S144 degree 2 poles (33.6376, -189.0359) (33.5561, -188.9717) (33.3535, -188.9297) (33.2473, -188.9297) knots 0 0 0 1 2 2 2
  spline S145 degree 2 poles (33.2473, -188.9297) (33.1041, -188.9297) (32.8348, -189.0162) (32.7039, -189.0977) knots 0 0 0 1 2 2 2
  spline S146 degree 2 poles (32.7039, -189.0977) (32.7015, -189.1421) (32.6965, -189.2261) (32.6965, -189.2903) knots 0 0 0 1 2 2 2
  spline S147 degree 2 poles (32.6965, -189.2903) (32.6965, -189.6065) (32.82, -189.9943) (32.9139, -190.0956) knots 0 0 0 1 2 2 2
  spline S148 degree 2 poles (32.9139, -190.0956) (33.0003, -190.1919) (33.1881, -190.2685) (33.2943, -190.2685) knots 0 0 0 1 2 2 2
  spline S149 degree 2 poles (33.2943, -190.2685) (33.5413, -190.2685) (33.8451, -189.9177) (33.8451, -189.567) knots 0 0 0 1 2 2 2
  point P0 (0, 0)
  constraints: 2 other
emboss "Emboss1" sketch "Sketch13" operation cut depth 2.54 direction (-1, 0, 0)